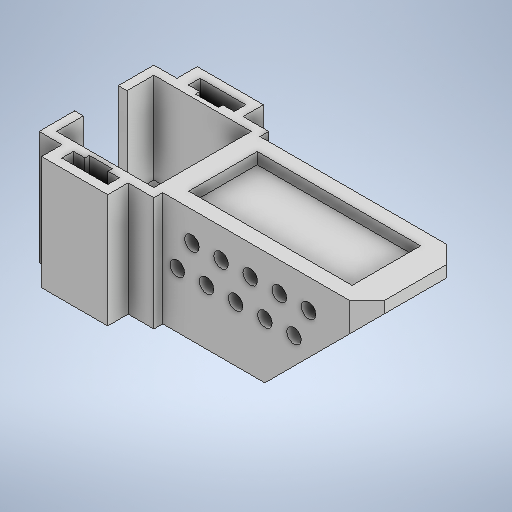
# Autodesk Inventor part: StepperMotorHolder
Saved by Autodesk Inventor 2027 (Build 310192060, 192F)
## iProperties
Created: 2026-06-30
Part Number: StepperMotorHolder
Material: Generic
Document SubType Name: Modeling
Designer: 13129
Density: 1 g/cm^3
Appearance: Default
Author: 13129
Autodesk Inventor part; units mm, degrees
ref_plane "YZ Plane" through (0, 0, 0) normal (1, 0, 0) x (0, 1, 0)
ref_plane "XZ Plane" through (0, 0, 0) normal (0, 1, 0) x (-1, 0, 0)
ref_plane "XY Plane" through (0, 0, 0) normal (0, 0, 1) x (1, 0, 0)
sketch "Sketch1" plane through (0, 0, 0) normal (0, 1, 0) x (-1, 0, 0)
  line L0 (0, 0) -> (50, 0)
  line L1 (50, 0) -> (50, -50)
  line L2 (50, -50) -> (0, -50)
  line L3 (0, -50) -> (0, 0)
  dimension "d0" = 50
  constraints: 8 end point, 2 equal length, 2 perpendicular, 1 horizontal
  measures "d0" distance of L0.start L0.end
extrude "Extrusion1" add sketch "Sketch1" along normal blind 10
sketch "Sketch2" plane through (0, 10, 0) normal (0, 1, 0) x (1, 0, 0)
  line L0 (0, 50) -> (-50, 50) construction
  line L1 (-50, 0) -> (0, 0) construction
  line L2 (0, 0) -> (0, 50) construction
  line L3 (-46.2, 46.2) -> (-3.8, 46.2)
  line L4 (-3.8, 46.2) -> (-3.8, 3.8)
  line L5 (-3.8, 3.8) -> (-46.2, 3.8)
  line L6 (0, 0) -> (-50, 0)
  line L7 (0, 0) -> (0, 50)
  line L8 (0, 50) -> (-50, 50)
  line L9 (-50, 50) -> (-50, 0) construction
  line L10 (-46.2, 34.5) -> (-46.2, 15.5)
  line L11 (-50, 50) -> (-50, 34.5)
  line L12 (-50, 34.5) -> (-46.2, 34.5)
  line L13 (-46.2, 34.5) -> (-46.2, 46.2)
  line L14 (-46.2, 0) -> (-50, 0)
  line L15 (-50, 0) -> (-50, 15.5)
  line L16 (-50, 15.5) -> (-46.2, 15.5)
  line L17 (-46.2, 15.5) -> (-46.2, 3.8)
  point P0 (0, 25)
  point P1 (-3.8, 25)
  point P2 (-25, 46.2)
  point P3 (-25, 50)
  point P4 (-46.2, 50)
  point P5 (-46.2, 25)
  dimension "d6" = 42.4
  dimension "d7" = 42.4
  dimension "d10" = 19
  dimension "d11" = 3.8
  constraints: 28 end point, 8 point on line, 5 midpoint, 5 perpendicular, 2 horizontal alignment, 2 vertical alignment, 1 collinear, 1 horizontal, 1 parallel, 1 vertical
  measures "d6" distance of L3.end L4.end
  measures "d7" distance of L4.end L5.end
  measures "d10" distance of L10.start L10.end
  measures "d11" distance between parallel lines of L4 L2
extrude "Extrusion2" add sketch "Sketch2" along normal blind 39.5 contours L13 L12 L11 L8 L7 L6 L15 L16 L17 L5 L4 L3
sketch "Sketch3" plane through (0, 49.5, 0) normal (0, 1, 0) x (1, 0, 0)
  line L0 (0, 0) -> (0, 50) construction
  line L1 (0, 50) -> (-50, 50) construction
  line L2 (-46.2, 46.2) -> (-3.8, 46.2) construction
  line L3 (-20, 50) -> (-20, 48.095)
  line L4 (-20, 48.095) -> (-30, 48.095)
  line L5 (-30, 48.095) -> (-30, 50)
  line L6 (-30, 50) -> (-20, 50)
  line L7 (0, 25) -> (-50, 25)
  line L8 (-50, 34.5) -> (-50, 15.5) construction
  line L9 (0, 0) -> (-50, 0) construction
  line L10 (-46.2, 3.8) -> (-3.8, 3.8) construction
  line L11 (-20, 0) -> (-20, 1.905)
  line L12 (-20, 1.905) -> (-30, 1.905)
  line L13 (-30, 1.905) -> (-30, 0)
  line L14 (-30, 0) -> (-20, 0)
  point P0 (-25, 48.095)
  point P1 (-25, 50)
  point P2 (-25, 1.905)
  point P3 (-25, 0)
  dimension "d12" = 1.905
  dimension "d13" = 10
  constraints: 22 end point, 6 symmetric about line, 4 midpoint, 4 point on line, 1 collinear, 1 parallel, 1 perpendicular, 1 vertical, 1 vertical alignment
  measures "d12" distance of L3.start L3.end
  measures "d13" distance of L3.end L4.end
extrude "Extrusion3" cut sketch "Sketch3" against normal through all
sketch "Sketch4" plane through (0, 49.5, 0) normal (0, 1, 0) x (1, 0, 0)
  line L0 (-3.8, 46.2) -> (-3.8, 3.8) construction
  line L1 (0, 0) -> (0, 50) construction
  line L2 (0, 3.85) -> (88.9, 3.85)
  line L3 (88.9, 3.85) -> (88.9, 46.15)
  line L4 (88.9, 46.15) -> (0, 46.15)
  line L5 (0, 3.85) -> (0, 46.15)
  point P0 (-3.8, 25)
  point P1 (88.9, 25)
  dimension "d16" = 88.9
  dimension "d17" = 42.3
  constraints: 8 end point, 2 midpoint, 2 perpendicular, 2 point on line, 1 collinear, 1 horizontal alignment, 1 vertical
  measures "d16" distance of L2.start L2.end
  measures "d17" distance between parallel lines of L4 L2
extrude "Extrusion4" add sketch "Sketch4" against normal blind 49.5
chamfer "Chamfer1" distance 7.62 angle 45 2 edges at (88.9, 24.75, -3.85) (88.9, 24.75, -46.15)
chamfer "Chamfer2" distance 44.45 angle 45 1 edges at (88.9, 0, -25)
sketch "Sketch5" plane through (0, 0, -3.85) normal (0, 0, 1) x (1, 0, 0)
  line L0 (0, 49.5) -> (81.28, 49.5) construction
  line L1 (0, 0) -> (0, 49.5) construction
  circle A0 centre (12.7, 36.8) radius 3.175
  circle A1 centre (25.4, 36.8) radius 3.175
  circle A2 centre (38.1, 36.8) radius 3.175
  circle A3 centre (50.8, 36.8) radius 3.175
  circle A4 centre (63.5, 36.8) radius 3.175
  circle A5 centre (6.35, 24.1) radius 3.175
  circle A6 centre (19.05, 24.1) radius 3.175
  circle A7 centre (31.75, 24.1) radius 3.175
  circle A8 centre (44.45, 24.1) radius 3.175
  circle A9 centre (57.15, 24.1) radius 3.175
  dimension "d26" = 6.35
  dimension "d27" = 12.7
  dimension "d28" = 12.7
  dimension "d29" = 12.7
  dimension "d30" = 12.7
  dimension "d31" = 12.7
  dimension "d32" = 12.7
  dimension "d33" = 6.35
  dimension "d34" = 12.7
  dimension "d35" = 12.7
  dimension "d36" = 12.7
  dimension "d37" = 12.7
  dimension "d38" = 12.7
  dimension "d39" = 6.35
  constraints: 10 centre point, 8 equal radius, 8 horizontal alignment
  measures "d26" diameter of A0
  measures "d27" distance of A1.centre A0.centre
  measures "d28" distance of A2.centre A1.centre
  measures "d29" distance of A3.centre A2.centre
  measures "d30" distance of A3.centre A4.centre
  measures "d31" distance from line of L0 A2.centre
  measures "d32" distance from line of L1 A0.centre
  measures "d33" diameter of A5
  measures "d34" distance of A6.centre A5.centre
  measures "d35" distance of A7.centre A6.centre
  measures "d36" distance of A8.centre A7.centre
  measures "d37" distance of A8.centre A9.centre
  measures "d38" vertical distance of A5.centre A0.centre
  measures "d39" distance from line of L1 A5.centre
extrude "Extrusion5" cut sketch "Sketch5" against normal through all
sketch "Sketch6" plane through (0, 49.5, 0) normal (0, 1, 0) x (1, 0, 0)
  line L0 (88.9, 11.47) -> (88.9, 38.53) construction
  line L1 (76.2, 10.0775) -> (5.08, 10.0775)
  line L2 (5.08, 10.0775) -> (5.08, 39.9225)
  line L3 (5.08, 39.9225) -> (76.2, 39.9225)
  line L4 (76.2, 39.9225) -> (76.2, 10.0775)
  point P0 (76.2, 25)
  point P1 (88.9, 25)
  dimension "d42" = 71.12
  dimension "d43" = 29.845
  dimension "d44" = 12.7
  constraints: 8 end point, 2 midpoint, 2 parallel, 1 horizontal, 1 horizontal alignment, 1 perpendicular
  measures "d42" distance of L2.end L3.end
  measures "d43" distance of L1.end L2.end
  measures "d44" distance between parallel lines of L0 L4
extrude "Extrusion6" cut sketch "Sketch6" against normal blind 5
sketch "Sketch7" plane through (0, 49.5, 0) normal (0, 1, 0) x (1, 0, 0)
  line L0 (-20, 50) -> (-20, 48.095) construction
  line L1 (-30, 48.095) -> (-30, 50) construction
  line L2 (-30, 50) -> (-50, 50) construction
  line L3 (-3.8, 46.2) -> (-3.8, 3.8) construction
  line L4 (-50, 0) -> (-30, 0) construction
  line L5 (-30, 0) -> (-30, 1.905) construction
  line L6 (-30, 1.905) -> (-20, 1.905) construction
  line L7 (-20, 0) -> (0, 0) construction
  line L8 (-34.98, -5.08) -> (-15.02, -5.08)
  line L9 (-34.98, 0) -> (-34.98, -5.08)
  line L10 (-15.02, 0) -> (-15.02, -5.08)
  line L11 (-11.21, 0) -> (-11.21, -8.89)
  line L12 (-11.21, -8.89) -> (-40, -8.89)
  line L13 (-40, -8.89) -> (-40, 0)
  line L14 (-50, 34.5) -> (-50, 15.5) construction
  line L15 (-50, 25) -> (-3.8, 25)
  line L16 (-15.02, 50) -> (-15.02, 55.08)
  line L17 (-34.98, 55.08) -> (-15.02, 55.08)
  line L18 (-34.98, 50) -> (-34.98, 55.08)
  line L19 (-11.21, 50) -> (-11.21, 58.89)
  line L20 (-11.21, 58.89) -> (-40, 58.89)
  line L21 (-40, 58.89) -> (-40, 50)
  line L22 (-50, 0) -> (-30, 0) construction
  line L23 (-40, 0) -> (-34.98, 0)
  line L24 (-15.02, 0) -> (-11.21, 0)
  line L25 (-11.21, 50) -> (-15.02, 50)
  line L26 (-34.98, 50) -> (-40, 50)
  point P0 (-25, 1.905)
  point P1 (-25, -5.08)
  point P2 (-25, 55.08)
  dimension "d49" = 5.08
  dimension "d50" = 19.96
  dimension "d52" = 3.81
  dimension "d53" = 3.81
  constraints: 37 end point, 9 symmetric about line, 5 midpoint, 4 collinear, 3 vertical, 2 parallel, 1 horizontal, 1 horizontal alignment, 1 perpendicular, 1 point on line, 1 vertical alignment
  measures "d49" distance of L9.start L8.start
  measures "d50" distance of L8.start L10.end
  measures "d52" distance between parallel lines of L11 L10
  measures "d53" distance between parallel lines of L12 L8
extrude "Extrusion7" add sketch "Sketch7" against normal blind 49.5
sketch "Sketch8" plane through (0, 0, 0) normal (0, -1, 0) x (1, 0, 0)
  line L0 (-50, -50) -> (-50, 0) construction
  line L1 (-22.06, -37.7) -> (-22.06, -12.3) construction
  line L2 (-28.41, -37.7) -> (-28.41, -12.3)
  line L3 (-15.71, -12.3) -> (-15.71, -37.7)
  arc A0 (-28.41, -37.7) -> (-15.71, -37.7) centre (-22.06, -37.7) ccw
  arc A1 (-15.71, -12.3) -> (-28.41, -12.3) centre (-22.06, -12.3) ccw
  point P0 (-22.06, -25)
  point P1 (-50, -25)
  dimension "d56" = 12.7
  dimension "d57" = 21.59
  dimension "d58" = 25.4
  constraints: 8 end point, 4 point on circle, 4 tangent, 2 centre point, 2 midpoint, 1 horizontal alignment, 1 parallel, 1 vertical
  measures "d56" distance between parallel lines of L2 L3
  measures "d57" distance between parallel lines of L0 L2
  measures "d58" distance of L3.start L3.end
extrude "Extrusion8" cut sketch "Sketch8" against normal blind 25.4
body "Solid1"
